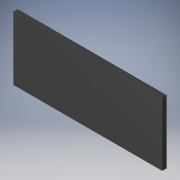
# Autodesk Inventor part: BA26
Saved by Autodesk Inventor 2017 (Build 210142000, 142)
## iProperties
Created: 2018-11-28
Part Number: BA26
Material: ABS Plastic
Document SubType Name: Modeling
Designer: Dell
Density: 1.06 g/cm^3
Appearance: Smooth - Black
Author: Dell
Autodesk Inventor part; units mm, degrees
ref_plane "YZ Plane" through (0, 0, 0) normal (1, 0, 0) x (0, 1, 0)
ref_plane "XZ Plane" through (0, 0, 0) normal (0, 1, 0) x (-1, 0, 0)
ref_plane "XY Plane" through (0, 0, 0) normal (0, 0, 1) x (1, 0, 0)
sketch "Sketch1" plane through (0, 0, 0) normal (0, 0, 1) x (1, 0, 0)
  line L0 (0, 0) -> (348, 0)
  line L1 (348, 0) -> (348, 148)
  line L2 (348, 148) -> (0, 148)
  line L3 (0, 148) -> (0, 0)
  dimension "d0" = 148
  dimension "d1" = 348
  constraints: 8 end point, 2 parallel, 1 horizontal, 1 perpendicular
  measures "d0" distance of L2.end L0.start
  measures "d1" distance of L1.end L2.end
extrude "Extrusion1" add sketch "Sketch1" along normal blind 10
body "Solid1"
